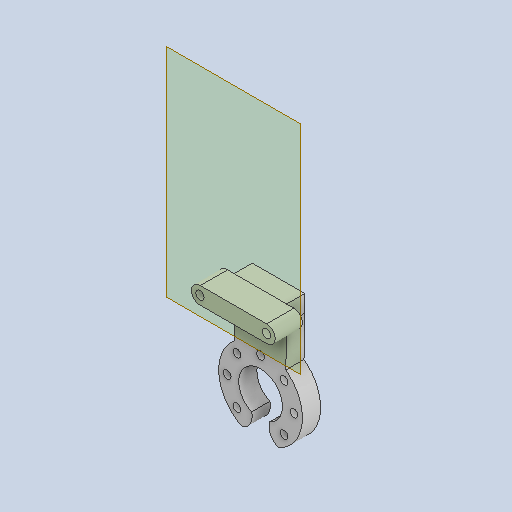
# Autodesk Inventor part: 0904_thigh_1
Saved by Autodesk Inventor 2024.3 (Build 283343000, 343)
## iProperties
Created: 2024-09-04
Part Number: 0904_thigh_1
Material: 일반
Document SubType Name: Modeling
Designer: gretc
Density: 1 g/cm^3
Appearance: 기본값
Author: gretc
Autodesk Inventor part; units mm, degrees
ref_plane "YZ Plane" through (0, 0, 0) normal (1, 0, 0) x (0, 1, 0)
ref_plane "XZ Plane" through (0, 0, 0) normal (0, 1, 0) x (-1, 0, 0)
ref_plane "XY Plane" through (0, 0, 0) normal (0, 0, 1) x (1, 0, 0)
ref_plane "작업 평면1" through (0, 0, -34) normal (0, 0, -1) x (-1, 0, 0)
sketch "스케치1" plane through (0, 0, -34) normal (0, 0, -1) x (-1, 0, 0)
  circle A0 centre (11, -47.8) radius 1.35 projected
  line L0 (15, -50.6) -> (-15, -50.6) projected
  line L1 (20.1, -44.6) -> (15, -50.6) projected
  line L2 (14.5, -40.1003) -> (14.5, -43) projected
  line L3 (8.25, -45) -> (-8.25, -45) projected
  line L4 (13.5, -39.75) -> (11.5, -39.75) projected
  arc A1 (11.5, -39.75) -> (9.25, -42) centre (11.5, -42) ccw projected
  line L5 (9.25, -42) -> (9.25, -44) projected
  arc A2 (8.25, -45) -> (9.25, -44) centre (8.25, -44) ccw projected
  line L6 (8.25, -45) -> (-8.25, -45) projected
  arc A3 (-9.25, -44) -> (-8.25, -45) centre (-8.25, -44) ccw projected
  line L7 (-9.25, -44) -> (-9.25, -42) projected
  arc A4 (-9.25, -42) -> (-11.5, -39.75) centre (-11.5, -42) ccw projected
  line L8 (-11.5, -39.75) -> (-13.5, -39.75) projected
  arc A5 (-14.5, -38.75) -> (-13.5, -39.75) centre (-13.5, -38.75) ccw projected
  line L9 (-14.5, -38.75) -> (-14.5, 8.25) projected
  arc A6 (-13.5, 9.25) -> (-14.5, 8.25) centre (-13.5, 8.25) ccw projected
  line L10 (-13.5, 9.25) -> (-11.5, 9.25) projected
  arc A7 (-11.5, 9.25) -> (-9.25, 11.5) centre (-11.5, 11.5) ccw projected
  line L11 (-9.25, 11.5) -> (-9.25, 14.5) projected
  line L12 (-15, 14.5) -> (-9.25, 14.5) projected
  line L13 (-20.1, 8.5) -> (-15, 14.5) projected
  line L14 (-20.1, -44.6) -> (-20.1, 8.5) projected
  line L15 (-15, -50.6) -> (-20.1, -44.6) projected
  line L16 (15, -50.6) -> (-15, -50.6) projected
  line L17 (20.1, -44.6) -> (15, -50.6) projected
  line L18 (20.1, 8.5) -> (20.1, -44.6) projected
  line L19 (15, 14.5) -> (20.1, 8.5) projected
  line L20 (9.25, 14.5) -> (15, 14.5) projected
  line L21 (9.25, 14.5) -> (9.25, 11.5) projected
  arc A8 (9.25, 11.5) -> (11.5, 9.25) centre (11.5, 11.5) ccw projected
  line L22 (11.5, 9.25) -> (13.5, 9.25) projected
  arc A9 (14.5, 8.25) -> (13.5, 9.25) centre (13.5, 8.25) ccw projected
  line L23 (14.5, 8.25) -> (14.5, -38.75) projected
  arc A10 (13.5, -39.75) -> (14.5, -38.75) centre (13.5, -38.75) ccw projected
  circle A11 centre (17.3, 4) radius 1.35 projected
  circle A12 centre (17.3, -18) radius 1.35 projected
  circle A13 centre (11, -47.8) radius 1.35 projected
  circle A14 centre (-17.3, 4) radius 1.35 projected
  circle A15 centre (-17.3, -18) radius 1.35 projected
  circle A16 centre (-11, -47.8) radius 1.35 projected
  circle A17 centre (17.3, -40) radius 1.35 projected
  circle A18 centre (-17.3, -40) radius 1.35 projected
  arc A19 (12.5, -45) -> (14.5, -43) centre (12.5, -43) ccw projected
  circle A20 centre (-11, -47.8) radius 2.8
  circle A21 centre (11, -47.8) radius 2.8
  line L24 (11.1003, -45) -> (12.5, -45) projected
  line L25 (7.025, -45) -> (10.8997, -45) projected
  line L26 (11, -44.9421) -> (13.475, -46.3711) projected
  line L27 (8.525, -46.3711) -> (11, -44.9421) projected
  line L28 (-10.8997, -45) -> (-7.025, -45) projected
  line L29 (-12.5, -45) -> (-11.1003, -45) projected
  arc A22 (-14.5, -43) -> (-12.5, -45) centre (-12.5, -43) ccw projected
  line L30 (-14.5, -40.1003) -> (-14.5, -43) projected
  line L31 (8.525, -46.3711) -> (11, -44.9421) projected
  line L32 (0, -45) -> (-11, -45)
  point P0 (0, 0)
  point P1 (-11, -50.6)
  point P2 (11, -50.6)
  point P3 (10.8964, -45.0019)
  constraints: 2 coincident, 2 end point, 1 centre point, 1 horizontal, 1 midpoint, 1 point on line, 1 tangent, 3 other
extrude "돌출1" add sketch "스케치1" along normal blind 9 contours L0 A20 L28 L3 L25 A21 | A21 L27 L26 | A20 | A21 L27 | L26 A21 picked at (12.0795, -46.0007)
sketch "스케치2" plane through (0, 0, -43) normal (0, 0, -1) x (-1, 0, 0)
  line L0 (-11, -50.6) -> (11, -50.6) projected
  line L1 (-8.6133, -50.6) -> (-8.6133, -44.9997)
  line L2 (-8.6133, -44.9997) -> (8.7217, -44.9997)
  line L3 (8.7217, -44.9997) -> (8.7217, -50.6)
  line L4 (8.7217, -50.6) -> (-8.6133, -50.6)
  line L5 (0.0542, -50.6) -> (0.0542, -44.9997)
  circle A0 centre (-11, -47.8) radius 1.35 projected
  circle A1 centre (11, -47.8) radius 1.35 projected
  circle A2 centre (0, -75) radius 13.8 projected
  circle A3 centre (0, -75) radius 7.2 projected
  circle A4 centre (0, -86) radius 1.2812 projected
  circle A5 centre (-7.7782, -82.7782) radius 1.2812 projected
  circle A6 centre (-11, -75) radius 1.2812 projected
  circle A7 centre (-7.7782, -67.2218) radius 1.2812 projected
  circle A8 centre (0, -64) radius 1.2812 projected
  circle A9 centre (7.7782, -67.2218) radius 1.2812 projected
  circle A10 centre (11, -75) radius 1.2812 projected
  circle A11 centre (7.7782, -82.7782) radius 1.2812 projected
  line L6 (-8.6133, -50.6) -> (-8.3331, -64)
  line L7 (8.7217, -50.6) -> (8.7217, -64.3055)
  circle A12 centre (-7.7782, -82.7782) radius 5
  circle A13 centre (7.7782, -82.7782) radius 5
  point P0 (0, 0)
  point P1 (-5.9724, -87.4407)
  point P2 (-2.924, -81.5795)
  point P3 (2.924, -81.5795)
  point P4 (5.9724, -87.4407)
  dimension "d2" = 5.6003
  dimension "d3" = 8.6675
  dimension "d4" = 2.3867
  dimension "d5" = 10
  dimension "d6" = 10
  constraints: 14 end point, 2 centre point, 2 coincident, 2 midpoint, 2 parallel, 2 perpendicular, 2 point on circle, 1 point on line, 1 vertical
  measures "d2" distance between parallel lines of L2 L0
  measures "d3" distance between parallel lines of L5 L1
  measures "d4" distance from line of L1 A0.centre
  measures "d5" diameter of A12
  measures "d6" diameter of A13
extrude "돌출2" add sketch "스케치2" along normal blind 6 contours L1 L2 L5 L0 | L0 L7 A2 L6 | L5 L2 L3 L0 | A2 A13 A3 A12 | A12 A3 A2 | A2 A13 A3 picked at (-4.5311, -64.4559)
